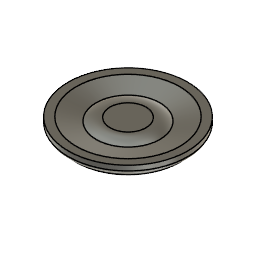
Helldivers Tacpad (Autodesk Fusion 360 archive; units mm, degrees)
design "2W Speaker"
Autodesk Fusion 360 part; units mm, degrees
sketch "Sketch1" plane through (0, 0, 0) normal (0, 0, 1) x (1, 0, 0)
  circle A0 centre (0, 0) radius 15
  circle A1 centre (0, 0) radius 8
  circle A2 centre (0, 0) radius 13
  line L0 (0, 0) -> (-5.494, 11.782)
  line L1 (0, 0) -> (13, 0) construction
  line L2 (0, 0) -> (5.494, 11.782)
  dimension "d1" = 30
  dimension "d2" = 16
  dimension "d3" = 26
  dimension "d4" = 115
  constraint coincident A0.centre A1.centre
  constraint horizontal L1
  constraint coincident A2 L0.end
  constraint coincident A2 L2.end
  measures "d1" diameter of A0
  measures "d2" diameter of A1
  measures "d3" diameter of A2
  measures "d4" angle of L0 L1
extrude "Extrude1" add sketch "Sketch1" along normal blind 5 contours A1 L0 L2 | A1 L0 L2 | A1 A2 L0 L2 picked at (-4.2011, 10.4954)
extrude "Extrude2" add sketch "Sketch1" along normal blind 3.5 contours A1 A2 L0 L2 picked at (11.2574, -1.0284)
extrude "Extrude3" add sketch "Sketch1" along normal blind 2.25
extrude "Extrude4" cut sketch "Sketch1" along normal blind 1 contours A1 L0 L2 | A1 L0 L2
chamfer "Chamfer1" distance 5 distance2 1 1 edges at (-7.4586, -2.8929, 0) measured on face at (12.6108, -0.7452, 0)
extrude "Extrude5" add 2 faces at (7.9602, 0.7965, 0.9999) (1.6626, -1.29, 1) along direction (0, 0, -1) blind 0.8
fillet "Fillet1" radius 8 1 edges at (-7.4586, 2.8929, 0.2)
fillet "Fillet2" radius 1 1 edges at (-13.9849, -5.4242, 2.25)
fillet "Fillet3" radius 0.6 1 edges at (0, -8, 5)
move_body "Move1" bodies 1 to x (-1, 0, 0) y (0, 1, 0) z (0, 0, -1) at (0, 0, 10)
